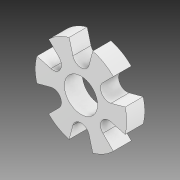
# Autodesk Inventor part: 1313_Drive Coil End_V2
Saved by Autodesk Inventor 2020 (Build 240168000, 168)
## iProperties
Created: 2019-10-22
Part Number: 1313_Drive Coil End_V2
Material: ABS Plastic
Document SubType Name: Modeling
Designer: RFLab
Density: 1.06 g/cm^3
Appearance: Smooth - White
Author: RFLab
Autodesk Inventor part; units mm, degrees
ref_plane "YZ Plane" through (0, 0, 0) normal (1, 0, 0) x (0, 1, 0)
ref_plane "XZ Plane" through (0, 0, 0) normal (0, 1, 0) x (-1, 0, 0)
ref_plane "XY Plane" through (0, 0, 0) normal (0, 0, 1) x (1, 0, 0)
sketch "Sketch12" plane through (0, 0, 0) normal (0, 0, 1) x (1, 0, 0)
  circle A0 centre (0, 0) radius 9.2
  circle A1 centre (0, 0) radius 25.3
  dimension "d46" = 18.4
  dimension "d47" = 50.6
  constraints: 2 centre point, 2 coincident
  measures "d46" diameter of A0
  measures "d47" diameter of A1
extrude "Extrusion12" add sketch "Sketch12" along normal blind 10
sketch "Sketch13" plane through (0, 0, 10) normal (0, 0, 1) x (1, 0, 0)
  circle A0 centre (0, 0) radius 25.3 projected
  circle A1 centre (0, 0) radius 9.2 projected
  line L0 (0, 0) -> (-6.5481, 24.4379) construction
  line L1 (0, 0) -> (6.5742, 24.5353) construction
  line L2 (0, 0) -> (0, 25.3) construction
  circle A2 centre (0, 0) radius 13.2 construction
  arc A3 (-4.4524, 16.6164) -> (4.4524, 16.6164) centre (0, 17.8094) ccw
  line L3 (-4.4524, 16.6164) -> (-6.5481, 24.4379)
  line L4 (4.4524, 16.6164) -> (6.5742, 24.5353)
  point P0 (6.5481, 24.4379)
  dimension "d50" = 30
  dimension "d51" = 15
  dimension "d52" = 4
  constraints: 10 end point, 4 point on circle, 2 centre point, 2 point on line, 2 tangent, 1 coincident, 1 collinear, 1 horizontal alignment, 1 vertical
  measures "d50" angle of L0 L1
  measures "d51" angle of L0 L2
  measures "d52" radial gap between concentric circles of A1 A2
extrude "Extrusion13" cut sketch "Sketch13" against normal through all contours A0 L4 A3 L3 picked at (-0.735, 19.4788)
pattern_circular "Circular Pattern3" count 6 over 360 about axis through (0, 0, 0) along (0, 0, 1) of "Extrusion13"
equation "\"d51\" = 0.5 * d50"
body "Solid2"
